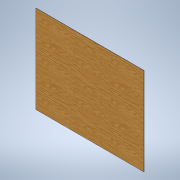
# Autodesk Inventor part: backboard
Saved by Autodesk Inventor 2022 (Build 260153000, 153)
## iProperties
Created: 2022-02-21
Part Number: backboard
Material: Plywood, Sheathing
Document SubType Name: Modeling
Designer: MarkP
Density: 0.552 g/cm^3
Appearance: Plywood - New
Author: MarkP
Autodesk Inventor part; units mm, degrees
ref_plane "YZ Plane" through (0, 0, 0) normal (1, 0, 0) x (0, 1, 0)
ref_plane "XZ Plane" through (0, 0, 0) normal (0, 1, 0) x (-1, 0, 0)
ref_plane "XY Plane" through (0, 0, 0) normal (0, 0, 1) x (1, 0, 0)
sketch "Sketch1" plane through (0, 0, 0) normal (0, 0, 1) x (1, 0, 0)
  line L0 (0, 0) -> (1500, 0)
  line L1 (1500, 0) -> (1500, 1220)
  line L2 (1500, 1220) -> (0, 1220)
  line L3 (0, 1220) -> (0, 0)
  dimension "d0" = 1500
  dimension "d1" = 1220
  constraints: 8 end point, 2 parallel, 1 horizontal, 1 perpendicular
  measures "d0" distance of L2.end L1.end
  measures "d1" distance of L1.end L0.end
extrude "Extrusion1" add sketch "Sketch1" along normal blind 3
body "Solid1"
